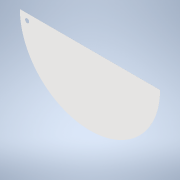
# Autodesk Inventor part: fllooor22
Saved by Autodesk Inventor 2021 (Build 250183000, 183)
## iProperties
Created: 2021-09-19
Part Number: fllooor22
Material: Stal nierdzewna
Document SubType Name: Konstrukcja blachowa
Designer: wojwo
Density: 8 g/cm^3
Sheet Metal Rule: Domyślny_mm
Appearance: Częściowo polerowana
Author: wojwo
Autodesk Inventor part; units mm, degrees
ref_plane "YZ Plane" through (0, 0, 0) normal (1, 0, 0) x (0, 1, 0)
ref_plane "XZ Plane" through (0, 0, 0) normal (0, 1, 0) x (-1, 0, 0)
ref_plane "XY Plane" through (0, 0, 0) normal (0, 0, 1) x (1, 0, 0)
sketch "Szkic1" plane through (0, 0, 0) normal (0, 0, 1) x (1, 0, 0)
  arc A0 (-870, 0) -> (870, 0) centre (0, 0) ccw
  line L0 (-870, 0) -> (870, 0)
  dimension "d0" = 1740
  measures "d0" diameter of A0
extrude "Płyta1" add sketch "Szkic1" along normal blind 3
sketch "Szkic2" plane through (0, 0, 3) normal (0, 0, 1) x (1, 0, 0)
  circle A0 centre (-780, -80) radius 25
  arc A1 (-870, 0) -> (870, 0) centre (0, 0) ccw projected
  dimension "d2" = 50
  dimension "d3" = 80
  dimension "d4" = 780
  constraints: 1 centre point
  measures "d2" diameter of A0
  measures "d3" vertical distance of A1.centre A0.centre
  measures "d4" horizontal distance of A1.centre A0.centre
extrude "Wyciągnięcie proste1" cut sketch "Szkic2" against normal blind 10
chamfer "Faza1" distance 2 angle 45 1 edges at (0, 0, 0)
equation "\"d1\" = Grubość"
equation "\"PromieńGięcia\" = Grubość"
equation "\"SzerokośćGięciaPodcięcia\" = Grubość"
equation "\"GłębokośćGięciaPodcięcia\" = 0.5 * Grubość"
equation "\"RozmiarPodcięciaNarożnika\" = 4 * Grubość"
equation "\"MinimalnaPozostałość\" = 2 * Grubość"
equation "\"PromieńPrzejścia\" = PromieńGięcia"
equation "\"Rozmiar_promienia_Jacobiego\" = PromieńGięcia"
equation "\"Wielk_odstępu\" = Grubość"
equation "\"Grubość\" = 3"
